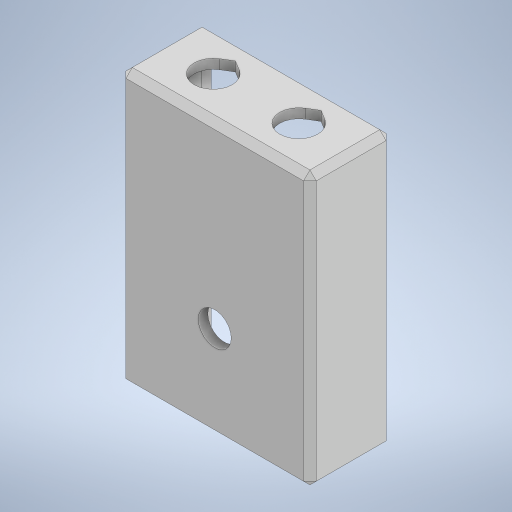
# Autodesk Inventor part: PotiBoxCase
Saved by Autodesk Inventor 2024.3 (Build 283343000, 343)
## iProperties
Created: 2025-03-30
Part Number: PotiBoxCase
Material: Generisch
Document SubType Name: Modeling
Designer: maxho
Density: 1 g/cm^3
Appearance: Vorgabe
Author: maxho
## iProperties of the stored document PotiBoxCase_3D-Druck.ipt
Created: 2025-03-30
Part Number: PotiBoxCase_3D-Druck
Material: Generisch
Document SubType Name: Modeling
Designer: maxho
Density: 1 g/cm^3
Appearance: Vorgabe
Author: maxho
Autodesk Inventor part; units mm, degrees
ref_plane "YZ Plane" through (0, 0, 0) normal (1, 0, 0) x (0, 1, 0)
ref_plane "XZ Plane" through (0, 0, 0) normal (0, 1, 0) x (-1, 0, 0)
ref_plane "XY Plane" through (0, 0, 0) normal (0, 0, 1) x (1, 0, 0)
sketch "Skizze1" plane through (0, 0, 0) normal (0, 1, 0) x (-1, 0, 0)
  line L0 (-30, -43) -> (30, -43)
  line L1 (30, -43) -> (30, 43)
  line L2 (30, 43) -> (-30, 43)
  line L3 (-30, 43) -> (-30, -43)
  line L4 (-30, -43) -> (30, 43) construction
  line L5 (30, -43) -> (-30, 43) construction
  point P0 (0, 0)
  dimension "d2" = 60
  dimension "d3" = 86
  constraints: 12 end point, 2 midpoint, 2 parallel, 1 horizontal, 1 perpendicular
  measures "d2" distance of L1.end L2.end
  measures "d3" distance of L0.end L1.end
extrude "Extrusion1" add sketch "Skizze1" along normal blind 26
shell "Wandung1" thickness 3 removed faces 1 at (-10, 26, -14.3333)
sketch "Skizze2" plane through (-30, 0, 43) normal (0, 0, 1) x (1, 0, 0)
  line L0 (0, 0) -> (60, 0) construction
  line L1 (60, 0) -> (60, 26) construction
  line L2 (0, 26) -> (60, 26) construction
  line L3 (0, 0) -> (0, 26) construction
  line L4 (3, 3) -> (57, 3) construction
  line L5 (3, 3) -> (3, 26) construction
  line L6 (57, 26) -> (3, 26) construction
  line L7 (57, 3) -> (57, 26) construction
  circle A0 centre (16.5, 13) radius 6
  circle A1 centre (43.5, 13) radius 6
  line L8 (3, 23) -> (57, 23) construction
  line L9 (3, 23) -> (30, 3) construction
  line L10 (30, 3) -> (57, 23) construction
  line L11 (19.5905, 18.1429) -> (16.5, 20)
  line L12 (16.5, 20) -> (13.4095, 18.1429)
  line L13 (46.5905, 18.1429) -> (43.5, 20)
  line L14 (43.5, 20) -> (40.4095, 18.1429)
  point P0 (30, 0)
  dimension "d5" = 12
  dimension "d19" = 3
  dimension "d20" = 7
  constraints: 14 end point, 4 point on circle, 4 tangent, 3 midpoint, 2 centre point, 2 point on line, 2 vertical alignment, 1 equal radius, 1 horizontal alignment, 1 perpendicular
  measures "d5" diameter of A0
  measures "d19" distance between parallel lines of L2 L8
  measures "d20" distance of A0.centre L11.end
extrude "Extrusion2" cut sketch "Skizze2" against normal up to surface (3 mm away)
sketch "Skizze3" plane through (0, 0, 0) normal (0, -1, 0) x (1, 0, 0)
  line L0 (-30, -43) -> (-30, 43) construction
  line L1 (30, -43) -> (-30, -43) construction
  line L2 (30, 43) -> (30, -43) construction
  line L3 (-30, 43) -> (30, 43) construction
  line L4 (-27, -40) -> (-27, 40) construction
  line L5 (-27, 40) -> (27, 40) construction
  line L6 (27, 40) -> (27, -40) construction
  line L7 (27, -40) -> (-27, -40) construction
  circle A0 centre (0, -13.3333) radius 5.205
  line L8 (0, -40) -> (0, -13.3333) construction
  line L9 (0, -13.3333) -> (0, 13.3333) construction
  line L10 (0, 13.3333) -> (0, 40) construction
  point P0 (0, 0)
  dimension "d8" = 10.41
  constraints: 6 end point, 2 collinear, 2 midpoint, 1 centre point, 1 point on line, 1 vertical
  measures "d8" diameter of A0
extrude "Extrusion3" cut sketch "Skizze3" against normal through all
sketch "Skizze4" plane through (30, 0, -43) normal (0, 0, -1) x (-1, 0, 0)
  line L0 (0, 0) -> (60, 0) construction
  line L1 (60, 0) -> (60, 26) construction
  line L2 (0, 26) -> (60, 26) construction
  line L3 (0, 0) -> (0, 26) construction
  line L4 (3, 3) -> (57, 3) construction
  line L5 (24.795, 3) -> (35.205, 3) construction
  line L6 (57, 3) -> (3, 3) construction
  line L7 (3, 3) -> (57, 3) construction
  line L8 (57, 3) -> (57, 26) construction
  line L9 (3, 3) -> (3, 26) construction
  line L10 (57, 26) -> (58.2426, 23) construction
  line L11 (58.2426, 23) -> (1.7574, 23) construction
  line L12 (1.7574, 23) -> (3, 26) construction
  line L13 (57.1082, 26) -> (58.3923, 22.9)
  line L14 (58.3923, 22.9) -> (1.6077, 22.9)
  line L15 (1.6077, 22.9) -> (2.8918, 26)
  line L16 (2.8918, 26) -> (57.1082, 26)
  line L17 (60, 26) -> (0, 26) projected
  point P0 (30, 0)
  point P1 (30, 26)
  point P2 (30, 23)
  point P3 (30, 26)
  dimension "d11" = 3
  dimension "d12" = 22.5
  dimension "d13" = 0.1
  constraints: 14 end point, 4 midpoint, 1 collinear, 1 horizontal, 1 vertical alignment, 2 other
  measures "d11" distance between parallel lines of L2 L11
  measures "d12" angle of L10 L8
  measures "d13" distance between parallel lines of L10 L13
extrude "Extrusion4" cut sketch "Skizze4" against normal up to surface (83 mm away)
chamfer "Fasen1" distance 2 angle 45 13 edges at (-30, 13, -43) (-30, 0, 0) (0, 0, -43) (30, 13, -43) (30, 0, 0) (0, 0, 43) (-30, 13, 43) (30, 13, 43) (-30, 26, 0) (0, 26, 43) (30, 26, 0) (28.5541, 26, -43) (-28.5541, 26, -43)
equation "\"d2\" = PotiBoxInnerWidth + 2 * PotiBoxThickness"
equation "\"d3\" = PotiBoxInnerLength + 2 * PotiBoxThickness"
equation "\"d0\" = PotiBoxInnerHeight + 2 * PotiBoxThickness"
equation "\"d4\" = PotiBoxThickness"
equation "\"d5\" = ConnectorDiameter"
equation "\"d19\" = PotiBoxThickness"
equation "\"d8\" = PotiDiameter"
equation "\"d11\" = PotiBoxThickness"
equation "\"d13\" = Clearance"
equation "\"PotiBoxInnerWidth\" = 54"
equation "\"PotiBoxThickness\" = 3"
equation "\"PotiBoxInnerLength\" = 80"
equation "\"PotiBoxInnerHeight\" = 20"
equation "\"ConnectorDiameter\" = 12"
equation "\"PotiDiameter\" = 10.41"
equation "\"Clearance\" = 0.1"
